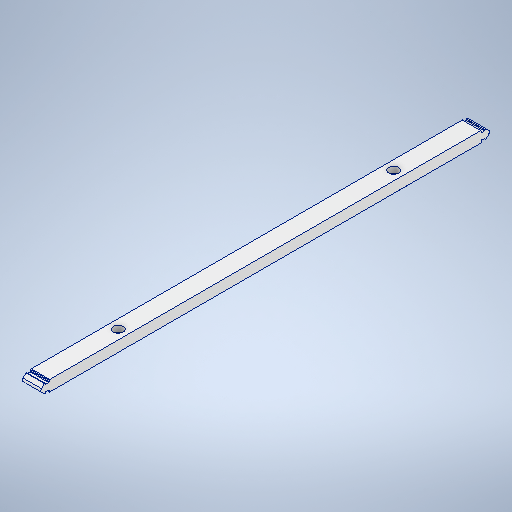
# Autodesk Inventor part: Support Rod
Saved by Autodesk Inventor 2025 (Build 290162000, 162)
## iProperties
Created: 2025-06-12
Part Number: Support Rod
Material: Aluminum 6061
Document SubType Name: Modeling
Designer: Caleb Fangmeier
Density: 2.7 g/cm^3
Appearance: Aluminum - Flat
Author: Caleb Fangmeier
Autodesk Inventor part; units mm, degrees
ref_plane "YZ Plane" through (0, 0, 0) normal (1, 0, 0) x (0, 1, 0)
ref_plane "XZ Plane" through (0, 0, 0) normal (0, 1, 0) x (-1, 0, 0)
ref_plane "XY Plane" through (0, 0, 0) normal (0, 0, 1) x (1, 0, 0)
sketch "Sketch1" plane through (0, 0, 0) normal (0, 0, 1) x (1, 0, 0)
  line L0 (8.5, -5) -> (-8.5, -5)
  line L1 (-8.5, -5) -> (-8.5, 5)
  line L2 (-8.5, 5) -> (8.5, 5)
  line L3 (8.5, 5) -> (8.5, -5)
  line L4 (8.5, -5) -> (-8.5, 5) construction
  line L5 (-8.5, -5) -> (8.5, 5) construction
  point P0 (0, 0)
  dimension "d0" = 17
  dimension "d1" = 10
  constraints: 12 end point, 2 midpoint, 2 parallel, 1 horizontal, 1 perpendicular
  measures "d0" distance of L1.end L2.end
  measures "d1" distance of L0.end L1.end
extrude "Extrusion1" add sketch "Sketch1" along normal blind 207.8
sketch "Sketch2" plane through (8.5, -5, 0) normal (1, 0, 0) x (0, 0, -1)
  line L0 (0, 10) -> (-207.8, 10) projected
  line L1 (-199.3, 10) -> (-199.3, 8)
  line L2 (-199.3, 8) -> (-202.8, 8)
  line L3 (-202.8, 8) -> (-202.8, 10)
  line L4 (-202.8, 10) -> (-207.8, 5)
  line L5 (-207.8, 5) -> (-202.8, 0)
  line L6 (-202.8, 0) -> (-202.8, 2)
  line L7 (-202.8, 2) -> (-199.3, 2)
  line L8 (-199.3, 2) -> (-199.3, 0)
  line L9 (0, 0) -> (-207.8, 0) projected
  line L10 (0, 10) -> (-207.8, 10) projected
  line L11 (-207.8, 0) -> (-207.8, 10) projected
  point P0 (0, 5)
  point P1 (-202.8, 0)
  point P2 (-202.8, 10)
  point P3 (-202.8, 10)
  dimension "d5" = 6
  dimension "d6" = 3.5
  dimension "d7" = 5
  constraints: 16 end point, 5 perpendicular, 4 equal length, 4 point on line, 2 vertical, 1 midpoint
  measures "d5" distance between parallel lines of L2 L7
  measures "d6" distance of L1.end L2.end
  measures "d7" horizontal distance of L4.end L2.end
extrude "Extrusion2" cut sketch "Sketch2" against normal through all
fillet "Fillet1" radius 0.5 8 edges at (0, 5, 199.3) (0, 3, 199.3) (0, 3, 202.8) (0, 5, 202.8) (0, -5, 202.8) (0, -3, 202.8) (0, -3, 199.3) (0, -5, 199.3)
fillet "Fillet2" radius 2 1 edges at (0, 0, 207.8)
mirror "Mirror2" about plane through (0, 0, 0) normal (0, 0, -1)
sketch "Sketch3" plane through (-8.5, -5, 198.8) normal (0, 1, 0) x (1, 0, 0)
  point P0 (8.5, 198.8)
  point P1 (8.5, 71.8)
  point P2 (8.5, 325.8)
  dimension "d12" = 254
  dimension "d13" = 127
  measures "d12" distance of point (8.5, 71.8) point (8.5, 325.8)
  measures "d13" distance of point (8.5, 71.8) point (8.5, 198.8)
hole "Hole1" at (0, -5, 127) at (0, -5, -127) direction (0, 1, 0) diameter 9 end through all countersink diameter 17.3 countersink angle 90 clearance for "Flat Head Machine Screw" size "M8" standard "Ansi Metric M Profile"
equation "\"d13\" = 0.5 * d12"
body "Solid1"
